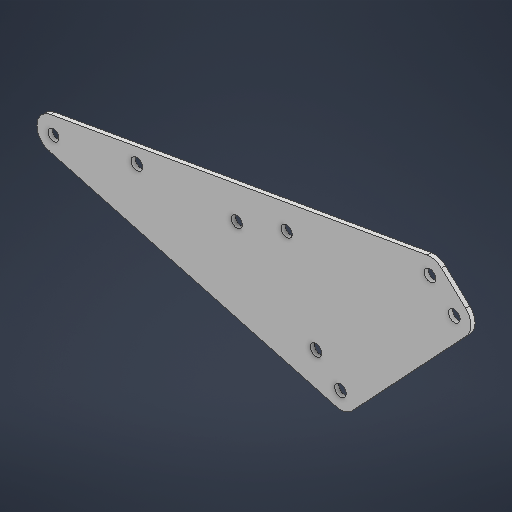
# Autodesk Inventor part: 1-Gearbox
Saved by Autodesk Inventor 2026.1 (Build 301233000, 233)
## iProperties
Created: 2025-08-06
Part Number: 1-Gearbox
Material: Generic
Document SubType Name: Modeling
Designer: roejo
Density: 1 g/cm^3
Appearance: Default
Author: roejo
Autodesk Inventor part; units mm, degrees
ref_plane "YZ Plane" through (0, 0, 0) normal (1, 0, 0) x (0, 1, 0)
ref_plane "XZ Plane" through (0, 0, 0) normal (0, 1, 0) x (-1, 0, 0)
ref_plane "XY Plane" through (0, 0, 0) normal (0, 0, 1) x (1, 0, 0)
sketch "Sketch1" plane through (0, 0, 0) normal (0, 0, 1) x (1, 0, 0)
  circle A0 centre (-44.4655, 8.6669) radius 2.2105
  circle A1 centre (-6.1332, 8.6669) radius 2.1083
  circle A2 centre (77.2932, 19.0809) radius 2.1977
  circle A3 centre (67.9723, 27.8207) radius 2.1977
  circle A4 centre (33.6091, -27.5374) radius 2.1977
  circle A5 centre (24.2854, -18.8006) radius 2.1977
  circle A6 centre (13.0328, 15.0558) radius 2.0955
  circle A7 centre (-76.4091, 2.2782) radius 2.0955
  arc A8 (-77.5153, 8.5311) -> (-78.0701, -3.8507) centre (-76.4091, 2.2782) ccw
  arc A9 (31.9481, -33.6663) -> (38.2426, -31.8793) centre (33.6091, -27.5374) ccw
  arc A10 (72.3158, 32.4529) -> (66.8661, 34.0736) centre (67.9723, 27.8207) ccw
  arc A11 (81.9268, 14.739) -> (81.6366, 23.7131) centre (77.2932, 19.0809) ccw
  line L0 (-78.0701, -3.8507) -> (31.9481, -33.6663)
  line L1 (38.2426, -31.8793) -> (81.9268, 14.739)
  line L2 (81.6366, 23.7131) -> (72.3158, 32.4529)
  line L3 (66.8661, 34.0736) -> (-77.5153, 8.5311)
  point P0 (0, 0)
  dimension "d0" = 4.191
  dimension "d1" = 4.191
  dimension "d3" = 12.7
  dimension "d5" = 12.7
  dimension "d6" = 12.7
  dimension "d7" = 12.7
  constraints: 12 centre point, 8 end point, 8 point on circle, 8 tangent, 4 coincident, 5 other
  measures "d0" diameter of A6
  measures "d1" diameter of A7
  measures "d3" diameter of A8
  measures "d5" diameter of A9
  measures "d6" diameter of A10
  measures "d7" diameter of A11
extrude "Extrusion1" add sketch "Sketch1" along normal blind 1.5875
body "Solid1"
